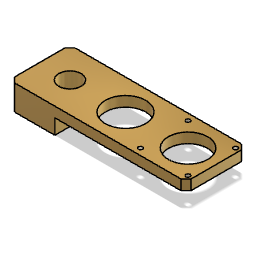
BC linear drive plate v6 (Autodesk Fusion 360 design; units mm, degrees)
Autodesk Fusion 360 part; units mm, degrees
sketch "Sketch1" plane through (0, 0, 0) normal (0, 1, 0) x (1, 0, 0)
  circle A0 centre (0, 0) radius 20
  circle A1 centre (-55, 0) radius 16 construction
  circle A2 centre (-55, 0) radius 11
  line L0 (0, 0) -> (-55, 0) construction
  line L1 (-85, 30) -> (90, 30)
  line L2 (90, 30) -> (90, -30)
  line L3 (90, -30) -> (-85, -30)
  line L4 (-85, -30) -> (-85, 30)
  line L5 (-40, 30) -> (-40, -30)
  line L6 (-66.3137, -11.3137) -> (-43.6863, 11.3137) construction
  line L7 (-66.3137, 11.3137) -> (-43.6863, -11.3137) construction
  line L8 (-55, 16) -> (-55, -16) construction
  line L9 (38.43, -23.57) -> (85.57, -23.57) construction
  line L10 (85.57, -23.57) -> (85.57, 23.57) construction
  line L11 (85.57, 23.57) -> (38.43, 23.57) construction
  line L12 (38.43, 23.57) -> (38.43, -23.57) construction
  line L13 (38.43, 23.57) -> (85.57, -23.57) construction
  circle A3 centre (62, 0) radius 19.5
  point P0 (-66.3137, 11.3137)
  point P1 (-55, 16)
  point P2 (-43.6863, 11.3137)
  point P3 (-43.6863, -11.3137)
  point P4 (-55, -16)
  point P5 (-66.3137, -11.3137)
  dimension "d1" = 32
  dimension "d2" = 22
  dimension "d3" = 55
  dimension "d4" = 40
  dimension "d5" = 60
  dimension "d6" = 30
  dimension "d7" = 90
  dimension "d8" = 15
  dimension "d9" = 45
  dimension "d20" = 47.14
  dimension "d22" = 39
  dimension "d27" = 62
  constraint coincident A0.centre L0.start
  constraint concentric A1 A2
  constraint coincident A1.centre A2.centre
  constraint horizontal L0
  constraint horizontal L1
  constraint vertical L2
  constraint horizontal L3
  constraint vertical L4
  constraint symmetric L0 L1 L3
  constraint coincident L1 L5.start
  constraint coincident L3 L5.end
  constraint perpendicular L3 L5
  constraint coincident A1 P5
  constraint coincident A1 P2
  constraint coincident A1 P0
  constraint coincident A1 P3
  constraint coincident A1 P1
  constraint coincident A1 P4
  constraint coincident A1.centre L6
  constraint perpendicular L6 L7
  constraint coincident A1.centre L7
  constraint vertical L8
  constraint coincident A1.centre L8
  constraint coincident P0 L7.start
  constraint coincident P1 L8.start
  constraint coincident P2 L6.end
  constraint coincident P3 L7.end
  constraint coincident P4 L8.end
  constraint coincident P5 L6.start
  constraint horizontal L9
  constraint vertical L10
  constraint horizontal L11
  constraint vertical L12
  constraint equal L9 L12
  constraint symmetric L0 L9 L11
  constraint midpoint L13 A3.centre
  measures "d1" diameter of A1
  measures "d2" diameter of A2
  measures "d3" distance of A0.centre A1.centre
  measures "d4" diameter of A0
  measures "d5" distance of L1.start L3.end
  measures "d6" distance of A1.centre L4
  measures "d7" distance of A0.centre L2
  measures "d8" distance of A1.centre L5
  measures "d9" angle of L7 L8
  measures "d20" distance of L9.start L9.end
  measures "d22" diameter of A3
  measures "d27" distance of A0.centre A3.centre
extrude "Extrude1" add sketch "Sketch1" along normal blind 25
extrude "Extrude3" cut sketch "Sketch1" along normal blind 15 contours L1 L2 L3 L5 | A3
hole "Hole1" at (-66.3137, 0, 11.3137) at (-55, 0, 16) at (-66.3137, 0, -11.3137) at (-55, 0, -16) at (-43.6863, 0, -11.3137) at (-43.6863, 0, 11.3137) direction (0, 1, 0) diameter 3.332 depth 15 tip angle 118
thread "Thread1" "ISO Metric profile 4.0 M4x0.7 6H" thread offset 0 thread depth 10
hole "Hole2" at (38.43, 0, 23.57) at (38.43, 0, -23.57) at (85.57, 0, 23.57) at (85.57, 0, -23.57) direction (0, 1, 0) diameter 4.234 depth 60 tip angle 118
thread "Thread2" "ISO Metric profile 5.0 M5x0.8 6H" thread offset 0 thread depth 10
chamfer "Chamfer1" distance 5 angle 45 4 edges at (-85, 12.5, -30) (-85, 12.5, 30) (90, 20, -30) (90, 20, 30)
